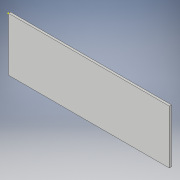
# Autodesk Inventor part: rev1 base large wall backplane
Saved by Autodesk Inventor 2017 (Build 210142000, 142)
## iProperties
Created: 2019-05-04
Part Number: rev1 base large wall backplane
Material: Generic
Document SubType Name: Modeling
Designer: Roman
Density: 1 g/cm^3
Appearance: Default
Author: Roman
Autodesk Inventor part; units mm, degrees
ref_plane "YZ Plane" through (0, 0, 0) normal (1, 0, 0) x (0, 1, 0)
ref_plane "XZ Plane" through (0, 0, 0) normal (0, 1, 0) x (-1, 0, 0)
ref_plane "XY Plane" through (0, 0, 0) normal (0, 0, 1) x (1, 0, 0)
sketch "Sketch1" plane through (0, 0, 0) normal (0, 0, 1) x (1, 0, 0)
  line L0 (0, 0) -> (1828.8, 0)
  line L1 (1828.8, 0) -> (1828.8, -609.6)
  line L2 (1828.8, -609.6) -> (0, -609.6)
  line L3 (0, -609.6) -> (0, 0)
  dimension "d0" = 1828.8
  dimension "d1" = 609.6
  constraints: 8 end point, 2 parallel, 1 horizontal, 1 perpendicular
  measures "d0" distance of L1.end L2.end
  measures "d1" distance of L0.end L1.end
extrude "Extrusion1" add sketch "Sketch1" along normal blind 25.4
sketch "Sketch2" plane through (0, 0, 25.4) normal (0, 0, 1) x (1, 0, 0)
  point P0 (0, 0)
body "Solid1"
